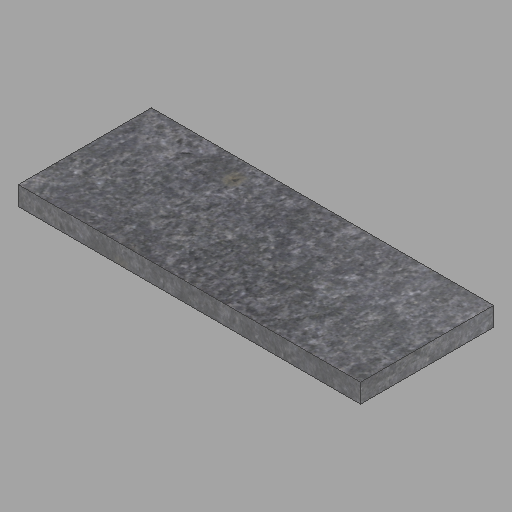
# Autodesk Inventor part: 2x14x36-18(2)
Saved by Autodesk Inventor 2023 (Build 270158000, 158)
## iProperties
Created: 2022-02-10
Part Number: 2x14x36-18(2)
Material: Granite, Cut, Polished
Document SubType Name: Modeling
Designer: awelt
Mass: 44599 g
Surface Area: 7793.53 cm^2
Volume: 16518.2 cm^3
Density: 2.7 g/cm^3
Appearance: Kasota SN sapphire
TEST: 0.0
Author: awelt
Autodesk Inventor part; units mm, degrees
ref_plane "YZ Plane" through (0, 0, 0) normal (1, 0, 0) x (0, 1, 0)
ref_plane "XZ Plane" through (0, 0, 0) normal (0, 1, 0) x (-1, 0, 0)
ref_plane "XY Plane" through (0, 0, 0) normal (0, 0, 1) x (1, 0, 0)
sketch "Sketch1" plane through (0, 0, 0) normal (1, 0, 0) x (0, 1, 0)
  line L0 (0, 0) -> (50.8, 0)
  line L1 (50.8, 0) -> (50.8, 355.6)
  line L2 (50.8, 355.6) -> (0, 355.6)
  line L3 (0, 355.6) -> (0, 0)
  dimension "d0" = 50.8
  dimension "d1" = 355.6
  constraints: 8 end point, 2 parallel, 1 horizontal, 1 perpendicular
  measures "d0" distance of L2.end L1.end
  measures "d1" distance of L1.end L0.end
extrude "Extrusion1" add sketch "Sketch1" along normal blind 914.4
body "Solid1"
